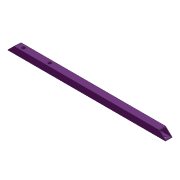
# Autodesk Inventor part: Part3
Saved by Autodesk Inventor 2012 (Build 160160000, 160)
## iProperties
Created: 2013-01-17
Part Number: Part3
Material: Aluminum-6061
Document SubType Name: Modeling
Designer: JesseK
Density: 2.71 g/cm^3
Mass: 237.993 g
Surface Area: 1113.56 cm^2
Volume: 87.8204 cm^3
Author: JesseK
Autodesk Inventor part; units mm, degrees
ref_plane "YZ Plane" through (0, 0, 0) normal (1, 0, 0) x (0, 1, 0)
ref_plane "XZ Plane" through (0, 0, 0) normal (0, 1, 0) x (-1, 0, 0)
ref_plane "XY Plane" through (0, 0, 0) normal (0, 0, 1) x (1, 0, 0)
sketch "Sketch1" plane through (0, 0, 0) normal (0, 0, 1) x (1, 0, 0)
  line L0 (0, 0) -> (609.6, 0)
  line L1 (609.6, 0) -> (609.6, 25.4)
  line L2 (609.6, 25.4) -> (0, 25.4)
  line L3 (0, 25.4) -> (0, 0)
  dimension "d0" = 25.4
  dimension "d1" = 609.6
  constraints: 8 end point, 2 parallel, 1 horizontal, 1 perpendicular
  measures "d0" distance of L2.end L0.start
  measures "d1" distance of L0.start L0.end
extrude "Extrusion1" add sketch "Sketch1" along normal blind 25.4
shell "Shell1" thickness 1.5875 removed faces 2 at (0, 16.9333, 8.4667) at (609.6, 8.4667, 8.4667)
sketch "Sketch2" plane through (0, 0, 25.4) normal (0, 0, 1) x (1, 0, 0)
  line L0 (0, 0) -> (0, 25.4) projected
  line L1 (609.6, 25.4) -> (609.6, 0) projected
  line L2 (0, 25.4) -> (609.6, 25.4) projected
  line L3 (0, 1.5875) -> (0, 25.4)
  line L4 (25.4, 25.4) -> (0, 1.5875)
  line L5 (0, 25.4) -> (25.4, 25.4)
  line L6 (584.2, 25.4) -> (609.6, 25.4)
  line L7 (609.6, 25.4) -> (609.6, 1.5875)
  line L8 (609.6, 1.5875) -> (584.2, 25.4)
  dimension "d5" = 25.4
  dimension "d6" = 1.5875
  dimension "d7" = 25.4
  dimension "d8" = 1.5875
  constraints: 12 end point, 4 point on line, 2 horizontal, 1 vertical
  measures "d5" distance of L0.end L4.start
  measures "d6" distance of L0.start L3.start
  measures "d7" distance of L6.start L1.start
  measures "d8" distance of L1.end L7.end
extrude "Extrusion2" cut sketch "Sketch2" against normal through all
sketch "Sketch3" plane through (0, 0, 0) normal (0, -1, 0) x (1, 0, 0)
  line L0 (0, 0) -> (0, 25.4) projected
  line L1 (0, 0) -> (609.6, 0) projected
  line L2 (609.6, 0) -> (609.6, 25.4) projected
  circle A0 centre (12.7, 12.7) radius 3.175
  circle A1 centre (596.9, 12.7) radius 3.175
  dimension "d11" = 12.7
  dimension "d12" = 12.7
  dimension "d13" = 6.35
  dimension "d14" = 12.7
  dimension "d15" = 12.7
  constraints: 2 centre point, 1 equal radius
  measures "d11" distance from line of L1 A0.centre
  measures "d12" distance from line of L0 A0.centre
  measures "d13" diameter of A0
  measures "d14" distance from line of L1 A1.centre
  measures "d15" distance from line of L2 A1.centre
extrude "Extrusion3" cut sketch "Sketch3" against normal through all
sketch "Sketch5" plane through (0, 0, 0) normal (0, -1, 0) x (1, 0, 0)
  circle A0 centre (12.7, 12.7) radius 3.175 projected
  line L0 (0, 0) -> (0, 25.4) projected
  circle A1 centre (47.625, 12.7) radius 3.175
  circle A2 centre (149.225, 12.7) radius 3.175
  line L1 (12.7, 12.7) -> (47.625, 12.7) construction
  line L2 (47.625, 12.7) -> (149.225, 12.7) construction
  dimension "d23" = 6.35
  dimension "d25" = 47.625
  dimension "d26" = 101.6
  constraints: 4 end point, 2 centre point, 2 horizontal, 1 equal radius
  measures "d23" diameter of A2
  measures "d25" distance from line of L1.end L0
  measures "d26" distance of L1.end L2.end
extrude "Extrusion5" cut sketch "Sketch5" against normal through all contours A1 | A2
sketch "Sketch6" plane through (25.4, 25.4, 0) normal (0, 1, 0) x (1, 0, 0)
  circle A0 centre (123.825, -12.7) radius 3.175 projected
  circle A1 centre (22.225, -12.7) radius 3.175 projected
  circle A2 centre (22.225, -12.7) radius 6.35
  circle A3 centre (123.825, -12.7) radius 6.35
  point P0 (-25.4, 0)
  dimension "d29" = 12.7
  dimension "d30" = 12.7
  constraints: 2 centre point, 2 coincident
  measures "d29" diameter of A3
  measures "d30" diameter of A2
extrude "Extrusion6" cut sketch "Sketch6" against normal up to next
body "Solid1"
